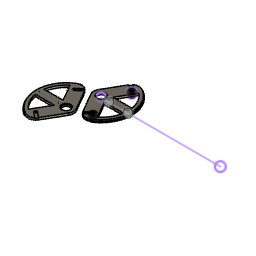
Writing Reducer (Autodesk Fusion 360 design; units mm, degrees)
Autodesk Fusion 360 part; units mm, degrees
note: some values were not read from the file. Set by a fixed rule: which sketch regions a step uses.
sketch "스케치1" plane through (0, 0, 0) normal (0, 0, 1) x (1, 0, 0)
  circle A0 centre (0, 0) radius 200 construction
  line L0 (0, 0) -> (800, 0) construction
  line L1 (0, 0) -> (100, 173.2051) construction
  line L2 (0, 0) -> (100, -173.2051) construction
  circle A1 centre (0, 0) radius 50 construction
  circle A2 centre (0, 0) radius 30
  circle A3 centre (75, 129.9038) radius 50 construction
  circle A4 centre (75, -129.9038) radius 50 construction
  line L3 (-43.3013, 25) -> (31.6987, 154.9038)
  line L4 (-43.3013, -25) -> (31.6987, -154.9038)
  arc A5 (100, -173.2051) -> (100, 173.2051) centre (0, 0) ccw
  circle A6 centre (75, 129.9038) radius 5
  circle A7 centre (75, 129.9038) radius 9 construction
  line L5 (31.6987, 154.9038) -> (69.1705, 123.0469)
  line L6 (80.8295, 136.7607) -> (43.3577, 168.6177)
  circle A8 centre (75, -129.9038) radius 5
  circle A9 centre (75, -129.9038) radius 9 construction
  line L7 (31.6987, -154.9038) -> (69.1705, -123.0469)
  line L8 (43.3577, -168.6177) -> (80.8295, -136.7607)
  arc A10 (-43.3013, 25) -> (-43.3013, -25) centre (0, 0) ccw
  circle A11 centre (0, 0) radius 180 construction
  circle A12 centre (75, -129.9038) radius 29 construction
  circle A13 centre (0, 0) radius 29 construction
  circle A14 centre (75, 129.9038) radius 29 construction
  line L9 (25.1147, 14.5) -> (113.939, -139.3481) construction
  line L10 (25.1147, -14.5) -> (113.939, 139.3481) construction
  line L11 (0.0002, 29) -> (177.6485, 29) construction
  line L12 (0, -29) -> (177.6485, -29) construction
  line L13 (50.2295, -29) -> (113.939, -139.3481)
  line L14 (50.2295, -29) -> (177.6485, -29)
  line L15 (50.2295, 29) -> (177.6485, 29)
  line L16 (50.2295, 29) -> (113.939, 139.3481)
  arc A15 (177.6485, 29) -> (113.939, 139.3481) centre (0, 0) ccw
  arc A16 (113.939, -139.3481) -> (177.6485, -29) centre (0, 0) ccw
  arc A17 (80.8295, -136.7607) -> (69.1705, -123.0469) centre (75, -129.9038) ccw
  arc A18 (31.6987, -154.9038) -> (43.3577, -168.6177) centre (75, -129.9038) ccw
  arc A19 (43.3577, -168.6177) -> (100, -173.2051) centre (75, -129.9038) ccw
  arc A20 (69.1705, 123.0469) -> (80.8295, 136.7607) centre (75, 129.9038) ccw
  arc A21 (43.3577, 168.6177) -> (31.6987, 154.9038) centre (75, 129.9038) ccw
  arc A22 (100, 173.2051) -> (43.3577, 168.6177) centre (75, 129.9038) ccw
  circle A23 centre (0, 0) radius 25
  circle A24 centre (0, 0) radius 205 construction
  line L17 (100, 173.2051) -> (102.5, 177.5352)
  line L18 (100, -173.2051) -> (102.5, -177.5352)
  arc A25 (102.5, -177.5352) -> (102.5, 177.5352) centre (0, 0) ccw
  dimension "d3" = 400
  dimension "d4" = 120
  dimension "d7" = 60
  dimension "d9" = 20
  dimension "d11" = 10
  dimension "d12" = 4
  dimension "d13" = 20
  dimension "d14" = 20
  dimension "d18" = 5
  dimension "d19" = 5
  constraint coincident A0.centre L0.start
  constraint horizontal L0
  constraint coincident A0 L1.end
  constraint coincident A0 L2.end
  constraint symmetric L0 L1 L2
  constraint coincident L1 A3.centre
  constraint coincident L1.end A3
  constraint coincident L2 A4.centre
  constraint coincident L2.end A4
  constraint equal A1 A3
  constraint equal A1 A4
  constraint coincident A1 L3.start
  constraint coincident A3 L3.end
  constraint tangent A3 L3
  constraint coincident A1 L4.start
  constraint coincident A4 L4.end
  constraint parallel L1 L3
  constraint parallel L2 L4
  constraint tangent A4 L4
  constraint tangent A4 A5
  constraint concentric A3 A6
  constraint concentric A3 A7
  constraint coincident A7 L5.end
  constraint tangent A7 L5
  constraint coincident A7 L6.start
  constraint coincident A3 L6.end
  constraint parallel L5 L6
  constraint tangent A7 L6
  constraint concentric A4 A8
  constraint concentric A4 A9
  constraint equal A6 A8
  constraint equal A7 A9
  constraint coincident A9 L7.end
  constraint tangent A9 L7
  constraint coincident A4 L8.start
  constraint coincident A9 L8.end
  constraint symmetric L0 L6 L8
  constraint tangent L4 A10
  constraint tangent L3 A10
  constraint concentric A5 A11
  constraint concentric A4 A12
  constraint concentric A10 A13
  constraint concentric A3 A14
  constraint equal A13 A14
  constraint equal A12 A13
  constraint coincident A13 L9.start
  constraint tangent A12 L9
  constraint tangent A13 L9
  constraint coincident A13 L10.start
  constraint tangent A14 L10
  constraint tangent A13 L10
  constraint coincident A11 L10.end
  constraint coincident A11 L9.end
  constraint coincident A13 L11.start
  constraint coincident A11 L11.end
  constraint coincident A13 L12.start
  constraint coincident A11 L12.end
  constraint tangent A13 L12
  constraint parallel L11 L12
  constraint coincident L12 L13.start
  constraint coincident L9 L13.start
  constraint coincident L11 L15.start
  constraint coincident L10 L15.start
  constraint tangent L8 A17
  constraint tangent L5 A20
  constraint tangent L3 A21
  constraint concentric A13 A23
  constraint concentric A2 A23
  constraint concentric A16 A24
  constraint coincident A24 L17.end
  constraint parallel L1 L17
  constraint coincident A24 L18.end
  constraint parallel L2 L18
  measures "d3" diameter of A0
  measures "d4" angle of L1 L2
  measures "d7" diameter of A2
  measures "d9" distance of A1 A2
  measures "d11" diameter of A6
  measures "d12" distance of A6 A7
  measures "d13" distance of A5 A11
  measures "d14" distance of A9 A12
  measures "d18" distance of A2 A23
  measures "d19" distance of A0 A24
sketch "스케치2" plane through (0, 0, 0) normal (0, 0, 1) x (1, 0, 0)
  circle A0 centre (75, 129.9038) radius 3
  circle A1 centre (75, 129.9038) radius 2.7 construction
  line L0 (73.4412, 132.6038) -> (76.5588, 132.6038)
  line L1 (76.5588, 132.6038) -> (78.1177, 129.9038)
  line L2 (78.1177, 129.9038) -> (76.5588, 127.2038)
  line L3 (76.5588, 127.2038) -> (73.4412, 127.2038)
  line L4 (73.4412, 127.2038) -> (71.8823, 129.9038)
  line L5 (71.8823, 129.9038) -> (73.4412, 132.6038)
  circle A2 centre (75, 129.9038) radius 5
  line L6 (0, 0) -> (800, 0)
  line L7 (73.4412, -127.2038) -> (71.8823, -129.9038)
  circle A3 centre (75, -129.9038) radius 3
  line L8 (76.5588, -132.6038) -> (78.1177, -129.9038)
  line L9 (76.5588, -127.2038) -> (73.4412, -127.2038)
  circle A4 centre (75, -129.9038) radius 2.7 construction
  line L10 (78.1177, -129.9038) -> (76.5588, -127.2038)
  line L11 (71.8823, -129.9038) -> (73.4412, -132.6038)
  line L12 (73.4412, -132.6038) -> (76.5588, -132.6038)
  circle A5 centre (50, 0) radius 2.7 construction
  line L13 (48.4412, 2.7) -> (46.8823, 0)
  line L14 (51.5588, 2.7) -> (48.4412, 2.7)
  circle A6 centre (50, 0) radius 3
  line L15 (46.8823, 0) -> (48.4412, -2.7)
  line L16 (51.5588, -2.7) -> (53.1177, 0)
  line L17 (48.4412, -2.7) -> (51.5588, -2.7)
  line L18 (53.1177, 0) -> (51.5588, 2.7)
  circle A7 centre (180, 0) radius 2.7 construction
  line L19 (178.4412, 2.7) -> (176.8823, 0)
  line L20 (181.5588, 2.7) -> (178.4412, 2.7)
  circle A8 centre (180, 0) radius 3
  line L21 (176.8823, 0) -> (178.4412, -2.7)
  line L22 (181.5588, -2.7) -> (183.1177, 0)
  line L23 (178.4412, -2.7) -> (181.5588, -2.7)
  line L24 (183.1177, 0) -> (181.5588, 2.7)
  circle A9 centre (75, -129.9038) radius 1.5
  circle A10 centre (50, 0) radius 1.5
  circle A11 centre (180, 0) radius 1.5
  circle A12 centre (75, 129.9038) radius 1.5
  point P0 (75, -129.9038)
  point P1 (50, 0)
  point P2 (180, 0)
  dimension "d38" = 6
  dimension "d39" = 5.4
  dimension "d40" = 120
  dimension "d41" = 120
  dimension "d47" = 3
  dimension "d48" = 3
  dimension "d49" = 3
  dimension "d50" = 3
  constraint concentric A0 A1
  constraint horizontal L0
  constraint parallel L0 L3
  constraint tangent A1 L0
  constraint tangent A1 L1
  constraint tangent A1 L2
  constraint tangent A1 L3
  constraint tangent A1 L4
  constraint tangent A1 L5
  constraint parallel L2 L5
  constraint parallel L1 L4
  constraint concentric A0 A2
  constraint symmetric A0 L6 A3
  constraint symmetric A1 L6 A4
  constraint symmetric L0.start L6 L11.end
  constraint symmetric L0.end L6 L8.start
  constraint symmetric L1.end L6 L8.end
  constraint symmetric L2.end L6 L9.start
  constraint symmetric L3.end L6 L7.start
  constraint symmetric L4.end L6 L7.end
  constraint symmetric A0.centre L6 P0
  constraint coincident L6 P1
  constraint coincident L6 P2
  constraint concentric A3 A9
  constraint concentric A6 A10
  constraint concentric A7 A11
  constraint concentric A2 A12
  measures "d38" diameter of A0
  measures "d39" diameter of A1
  measures "d40" angle of L3 L4
  measures "d41" angle of L0 L5
  measures "d47" diameter of A9
  measures "d48" diameter of A10
  measures "d49" diameter of A11
  measures "d50" diameter of A12
extrude "돌출1" add sketch "스케치1" along normal blind 5 contours A2 | L3 L4 A5 L5 L6 L7 L8 A10 A17 A19 A20 A22 | L5 L6 A20 A21 | L7 L8 A17 A18 | A5 L17 L18 A25 | A6 | A8 makes body 1
extrude "돌출2" add sketch "스케치1" along normal blind 9 separate body contours L3 L4 A5 L5 L6 L7 L8 A10 A17 A19 A20 A22 | A6 | A8 makes body 2 at (92.7025, 9.6667, 0) makes body 3 at (79.9938, 129.6546, 6) makes body 4 at (70.3926, -131.846, 6)
combine "결합1" operation add target body 1 tool bodies 2
combine "결합2" operation add target body 1 tool bodies 3
combine "결합3" operation add target body 1 tool bodies 4
extrude "돌출3" add sketch "스케치2" along normal blind 100 separate body contours L6 A10 | L6 A10 | L6 A11 | L6 A11 | A9 | A12 makes body 5 at (179.3831, 1.3673, 33.3333) makes body 6 at (73.9526, 128.83, 66.6667) makes body 7 at (49.3831, -1.3673, 66.6667) makes body 8 at (73.9526, -130.9776, 66.6667)
combine "결합4" operation cut target body 1 tool bodies 5
combine "결합5" operation cut target body 1 tool bodies 6
combine "결합6" operation cut target body 1 tool bodies 7
combine "결합7" operation cut target body 1 tool bodies 8
extrude "돌출4" add sketch "스케치2" along normal blind 3 separate body contours A0 L0 L1 L2 L3 L4 L5 | A0 L1 | A0 L2 | A0 L0 | A0 L3 | A0 L5 | A0 L4 | L6 L13 L14 A6 L18 A10 | L6 A6 L15 L16 L17 A10 | A6 L18 | A6 L16 | L13 A6 | A6 L15 | L14 A6 | A6 L17 | L6 L19 L20 A8 L24 A11 | L6 A8 L21 L22 L23 A11 | A8 L24 | A8 L22 | L19 A8 | A8 L21 | L20 A8 | A8 L23 | L7 A3 L8 L9 L10 L11 L12 | L7 A3 | A3 L9 | A3 L11 | A3 L10 | A3 L12 | A3 L8 makes body 9 at (179.9252, -2.9991, 1) makes body 10 at (74.9252, 126.9047, 1) makes body 11 at (50.373, -2.9767, 2) makes body 12 at (76.2339, -132.6383, 2)
extrude "돌출5" add sketch "스케치2" along normal blind 2 separate body contours A0 L0 L1 L2 L3 L4 L5 | A0 L1 L2 | A0 L0 L1 | A0 L2 L3 | A0 L0 L5 | A0 L3 L4 | A0 L4 L5 | L6 L13 L14 A6 L18 A10 | L6 A6 L15 L16 L17 A10 | L6 A6 L18 | L6 A6 L16 | L6 A6 L15 | L6 L13 A6 | L14 A6 L18 | A6 L16 L17 | L13 L14 A6 | A6 L15 L17 | L6 L19 L20 A8 L24 A11 | L6 A8 L21 L22 L23 A11 | L6 A8 L24 | L6 A8 L22 | L6 A8 L21 | L6 L19 A8 | L20 A8 L24 | A8 L22 L23 | L19 L20 A8 | A8 L21 L23 | L7 A3 L9 | L7 A3 L8 L9 L10 L11 L12 | L7 A3 L11 | A3 L9 L10 | A3 L11 L12 | A3 L8 L10 | A3 L8 L12 makes body 13 at (179.3831, 1.3673, 1.3333) makes body 14 at (73.9526, -130.9776, 1.3333) makes body 15 at (49.3157, -1.3348, 0.6667) makes body 16 at (73.9526, 128.83, 1.3333)
copy_body "CopyPasteBodies1" bodies 1 makes body 17
combine "결합8" operation cut target body 1 tool bodies 9
combine "결합9" operation cut target body 1 tool bodies 10
combine "결합10" operation cut target body 1 tool bodies 11
combine "결합11" operation cut target body 1 tool bodies 12
combine "결합12" operation cut target body 17 tool bodies 16
combine "결합13" operation cut target body 17 tool bodies 15
combine "결합14" operation cut target body 17 tool bodies 14
combine "결합15" operation cut target body 17 tool bodies 13
move_body "이동1" bodies 17 to x (1, 0, 0) y (0, 1, 0) z (0, 0, 1) at (350, 0, 0)
move_face "면 간격띄우기1" offset 5 12 faces at (384.3704, 102.6223, 9) (423.909, -126.24, 9) (423.8376, 133.5456, 9) (378.2216, 1.4904, 5) (416.0248, -146.7189, 5) (416.0248, 146.7189, 5) (34.3704, 102.6223, 9) (75.5328, -126.1183, 9) (78.8091, 129.5809, 9) (28.2216, 1.4904, 5) (66.0248, -146.7189, 5) (66.0248, 146.7189, 5) on bodies 1 17
move_body "이동2" bodies 17 to x (-1, 0, 0) y (0, -1, 0) z (0, 0, 1) at (300, -184.8076, 0)
equation "carbon_rod_D = 25 mm"
equation "carbon_rod_L = 400 mm"
equation "bearing_out = 60 mm"
equation "bearing_inner = 50 mm"
equation "d7 = bearing_out"
equation "thk = 20 mm"
equation "d9 = thk"
equation "rope_d = 4 mm"
equation "d12 = rope_d"
equation "d13 = thk"
equation "d14 = thk"
equation "thn = 5 mm"
equation "d18 = thn"
equation "d19 = thn"
equation "m3_hole = 3 mm"
equation "m3_nut_wid = 5.4 mm"
equation "m3_nut_height = 2 mm"
equation "m3_bolt_height = 3 mm"
equation "m3_bolt_width = 6 mm"
equation "error = 0.5 mm"
equation "d38 = m3_bolt_width"
equation "d39 = m3_nut_wid"
equation "d42 = thn"
equation "bearing_height = 8 mm"
equation "d45 = thn + bearing_height / 2"
equation "d47 = m3_hole"
equation "d48 = m3_hole"
equation "d49 = m3_hole"
equation "d50 = m3_hole"
equation "d53 = m3_bolt_height"
equation "d55 = m3_nut_height"
